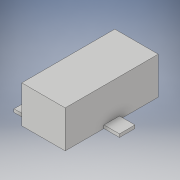
# Autodesk Inventor part: bc848
Saved by Autodesk Inventor 2019 (Build 230136000, 136)
## iProperties
Created: 2019-04-04
Part Number: bc848
Material: Generic
Document SubType Name: Modeling
Designer: jmc
Density: 1 g/cm^3
Appearance: Default
Author: jmc
Autodesk Inventor part; units mm, degrees
ref_plane "YZ Plane" through (0, 0, 0) normal (1, 0, 0) x (0, 1, 0)
ref_plane "XZ Plane" through (0, 0, 0) normal (0, 1, 0) x (-1, 0, 0)
ref_plane "XY Plane" through (0, 0, 0) normal (0, 0, 1) x (1, 0, 0)
sketch "Sketch1" plane through (0, 0, 0) normal (0, 1, 0) x (-1, 0, 0)
  line L0 (0.7, 1.5) -> (-0.7, 1.5)
  line L1 (-0.7, 1.5) -> (-0.7, -1.5)
  line L2 (-0.7, -1.5) -> (0.7, -1.5)
  line L3 (0.7, -1.5) -> (0.7, 1.5)
  line L4 (0.7, 1.5) -> (-0.7, -1.5) construction
  line L5 (-0.7, 1.5) -> (0.7, -1.5) construction
  point P0 (0, 0)
  dimension "d0" = 1.4
  dimension "d1" = 3
  constraints: 12 end point, 2 midpoint, 2 parallel, 1 horizontal, 1 perpendicular
  measures "d0" distance of L2.end L1.end
  measures "d1" distance of L1.end L0.end
extrude "Extrusion1" add sketch "Sketch1" along normal blind 1.2
sketch "Sketch2" plane through (0, 0, 0) normal (0, -1, 0) x (1, 0, 0)
  line L0 (0.7, 1.5) -> (0.7, -1.5) projected
  line L1 (-0.7, 1.25) -> (-1.2, 1.25)
  line L2 (-1.2, 1.25) -> (-1.2, 0.75)
  line L3 (-1.2, 0.75) -> (-0.7, 0.75)
  line L4 (-0.7, 1.25) -> (-1.2, 0.75) construction
  line L5 (-1.2, 1.25) -> (-0.7, 0.75) construction
  line L6 (-0.7, -0.75) -> (-1.2, -0.75)
  line L7 (-1.2, -0.75) -> (-1.2, -1.25)
  line L8 (-1.2, -1.25) -> (-0.7, -1.25)
  line L9 (-0.7, -1.25) -> (-0.7, -0.75)
  line L10 (-0.7, -0.75) -> (-1.2, -1.25) construction
  line L11 (-1.2, -0.75) -> (-0.7, -1.25) construction
  line L12 (1.2, 0.25) -> (0.7, 0.25)
  line L13 (0.7, 0.25) -> (0.7, -0.25)
  line L14 (0.7, -0.25) -> (1.2, -0.25)
  line L15 (1.2, -0.25) -> (1.2, 0.25)
  line L16 (1.2, 0.25) -> (0.7, -0.25) construction
  line L17 (0.7, 0.25) -> (1.2, -0.25) construction
  line L18 (-0.7, 1.25) -> (-0.7, 0.75)
  point P0 (0, 0)
  point P1 (-0.7, 0)
  point P2 (-0.95, 1)
  point P3 (-0.95, -1)
  point P4 (0.95, 0)
  dimension "d5" = 0.5
  dimension "d6" = 0.5
  dimension "d7" = 0.5
  dimension "d8" = 0.5
  dimension "d9" = 0.5
  dimension "d10" = 0.5
  constraints: 36 end point, 6 midpoint, 5 parallel, 3 horizontal, 3 perpendicular, 1 collinear, 1 vertical
  measures "d5" distance of L3.end L2.end
  measures "d6" distance of L2.end L1.end
  measures "d7" distance of L8.end L7.end
  measures "d8" distance of L7.end L6.end
  measures "d9" distance of L14.end L13.end
  measures "d10" distance of L13.end L12.end
extrude "Extrusion2" add sketch "Sketch2" against normal blind 0.1
body "Solid1"
